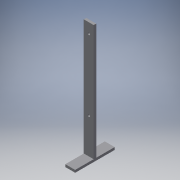
# Autodesk Inventor part: cPvcSupport
Saved by Autodesk Inventor 2016 SP1 (Build 200210100, 210)
## iProperties
Created: 2016-01-12
Part Number: cPvcSupport
Material: Generic
Document SubType Name: Modeling
Designer: steele
Density: 1 g/cm^3
Appearance: Default
Author: steele
Autodesk Inventor part; units mm, degrees
ref_plane "YZ Plane" through (0, 0, 0) normal (1, 0, 0) x (0, 1, 0)
ref_plane "XZ Plane" through (0, 0, 0) normal (0, 1, 0) x (-1, 0, 0)
ref_plane "XY Plane" through (0, 0, 0) normal (0, 0, 1) x (1, 0, 0)
sketch "Sketch1" plane through (0, 0, 0) normal (0, 0, 1) x (1, 0, 0)
  line L0 (0, 0) -> (12.7, 0)
  line L1 (12.7, 0) -> (12.7, 304.8)
  line L2 (12.7, 304.8) -> (0, 304.8)
  line L3 (0, 304.8) -> (0, 0) construction
  line L4 (0, 0) -> (-12.7, 0)
  line L5 (-12.7, 0) -> (-12.7, 304.8)
  line L6 (-12.7, 304.8) -> (0, 304.8)
  circle A0 centre (0, 279.4) radius 3.175
  dimension "d0" = 304.8
  dimension "d1" = 25.4
  dimension "d2" = 25.4
  dimension "d3" = 6.35
  dimension "d4" = 279.4
  constraints: 14 end point, 2 symmetric about line, 1 centre point, 1 horizontal, 1 parallel, 1 point on line, 1 vertical
  measures "d0" distance between parallel lines of L0 L2
  measures "d1" distance of L0.end L5.start
  measures "d2" distance of L1.end L6.start
  measures "d3" diameter of A0
  measures "d4" distance of A0.centre L0.start
extrude "Extrusion1" add sketch "Sketch1" along normal mid plane 6.35
sketch "Sketch2" plane through (0, 0, 0) normal (0, 0, 1) x (1, 0, 0)
  line L0 (-12.7, 0) -> (12.7, 0) projected
  line L1 (-12.7, 0) -> (12.7, 0)
  line L2 (12.7, 0) -> (12.7, 6.35)
  line L3 (12.7, 0) -> (12.7, 304.8) projected
  line L4 (-12.7, 304.8) -> (-12.7, 0) projected
  line L5 (-12.7, 6.35) -> (-12.7, 0)
  line L6 (-12.7, 6.35) -> (12.7, 6.35)
  point P0 (0, 0)
  dimension "d7" = 6.35
  constraints: 8 end point, 2 collinear, 2 point on line, 1 horizontal
  measures "d7" distance between parallel lines of L6 L0
extrude "Extrusion2" add sketch "Sketch2" along normal mid plane 101.6
sketch "Sketch3" plane through (0, 0, 3.175) normal (0, 0, 1) x (1, 0, 0)
  circle A0 centre (0, 97.3407) radius 3.175
  line L0 (-12.7, 0) -> (12.7, 0) projected
  point P0 (0, 0)
  dimension "d10" = 97.3407
  dimension "d11" = 6.35
  constraints: 1 centre point
  measures "d10" distance from line of A0.centre L0
  measures "d11" diameter of A0
extrude "Extrusion3" cut sketch "Sketch3" against normal through all
equation "\"d0\" = catapultSideHeight"
equation "\"d1\" = catapultSideWidth"
equation "\"d2\" = catapultTopWidth"
equation "\"d3\" = catpultSideHoleDiam"
equation "\"d4\" = catapultSideHoleHeight"
equation "\"d5\" = catapultSideDepth"
equation "\"d7\" = catapultSideDepth"
equation "\"d8\" = catapultSupportWidth"
equation "\"d11\" = catpultSideHoleDiam"
equation "\"catapultSideHeight\" = 304.8"
equation "\"catapultSideWidth\" = 25.4"
equation "\"catapultSideDepth\" = 6.35"
equation "\"catpultSideHoleDiam\" = 6.35"
equation "\"catapultTopWidth\" = 25.4"
equation "\"catapultSupportWidth\" = 101.6"
equation "\"catapultSupportPullyHeight\" = 152.4"
equation "\"catapultSideHoleHeight\" = 279.4"
body "Solid1"
